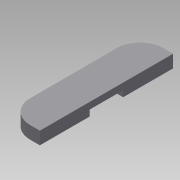
# Autodesk Inventor part: pig_wings
Saved by Autodesk Inventor 2015 (Build 190159000, 159)
## iProperties
Created: 2016-04-29
Part Number: pig_wings
Material: Generic
Document SubType Name: Modeling
Designer: Luke Good
Density: 1 g/cm^3
Appearance: Default
Author: Luke Good
Autodesk Inventor part; units mm, degrees
ref_plane "YZ Plane" through (0, 0, 0) normal (1, 0, 0) x (0, 1, 0)
ref_plane "XZ Plane" through (0, 0, 0) normal (0, 1, 0) x (-1, 0, 0)
ref_plane "XY Plane" through (0, 0, 0) normal (0, 0, 1) x (1, 0, 0)
sketch "Sketch1" plane through (0, 0, 0) normal (0, 1, 0) x (-1, 0, 0)
  line L0 (-2.6035, 25.4) -> (-6.2865, 25.4)
  line L1 (-6.2865, 25.4) -> (-6.2865, -25.4)
  line L2 (-6.2865, -25.4) -> (-2.6035, -25.4)
  line L3 (6.2865, -16.51) -> (6.2865, 16.51)
  line L4 (6.2865, 25.4) -> (-6.2865, -25.4) construction
  line L5 (-6.2865, 25.4) -> (6.2865, -25.4) construction
  arc A0 (6.2865, 16.51) -> (-2.6035, 25.4) centre (-2.6035, 16.51) ccw
  arc A1 (-2.6035, -25.4) -> (6.2865, -16.51) centre (-2.6035, -16.51) ccw
  point P0 (0, 0)
  dimension "d0" = 12.573
  dimension "d1" = 50.8
  dimension "d2" = 8.89
  constraints: 12 end point, 4 point on circle, 4 point on line, 4 tangent, 2 centre point, 2 midpoint, 2 parallel, 1 equal radius, 1 horizontal, 1 perpendicular
  measures "d0" distance of L5.end L1.end
  measures "d1" distance of L1.end L0.end
  measures "d2" radius of A0
extrude "Extrusion1" add sketch "Sketch1" along normal blind 4.826
sketch "Sketch2" plane through (6.2865, 0, 25.4) normal (1, 0, 0) x (0, 0, -1)
  line L0 (20.3835, 2.1639) -> (30.4165, 2.1639)
  line L1 (25.4, 0) -> (20.3835, 2.1639) construction
  line L2 (25.4, 0) -> (30.4165, 2.1639) construction
  line L3 (50.8, 0) -> (0, 0) projected
  line L4 (20.066, 2.1639) -> (20.066, 2.3009)
  line L5 (20.066, 2.3009) -> (30.734, 2.3009)
  line L6 (30.734, 2.3009) -> (30.734, 2.1639)
  line L7 (25.4, 0) -> (20.066, 2.3009) construction
  line L8 (25.4, 0) -> (30.734, 2.3009) construction
  line L9 (30.734, -2.3009) -> (30.4165, -2.3009)
  line L10 (20.3835, -2.3009) -> (20.066, -2.3009)
  line L11 (20.066, 2.3009) -> (19.05, 2.3009)
  line L12 (19.05, 2.3009) -> (19.05, 0)
  line L13 (30.734, 2.3009) -> (31.75, 2.3009)
  line L14 (31.75, 2.3009) -> (31.75, 0)
  point P0 (20.3835, 0)
  point P1 (30.4165, 0)
  point P2 (20.066, 0)
  point P3 (30.734, 0)
  constraints: 30 end point, 6 point on line, 3 horizontal, 3 parallel, 2 perpendicular, 2 vertical, 8 other
extrude "Extrusion2" cut sketch "Sketch2" against normal blind 12.7
body "Solid1"
